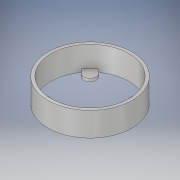
# Autodesk Inventor part: aluminumMount
Saved by Autodesk Inventor 2017 (Build 210142000, 142)
## iProperties
Created: 2016-10-18
Part Number: aluminumMount
Material: Aluminum 6061-AHC
Document SubType Name: Modeling
Designer: cflannery
Density: 2.7 g/cm^3
Appearance: Aluminum - Dark
Author: cflannery
Autodesk Inventor part; units mm, degrees
ref_plane "YZ Plane" through (0, 0, 0) normal (1, 0, 0) x (0, 1, 0)
ref_plane "XZ Plane" through (0, 0, 0) normal (0, 1, 0) x (-1, 0, 0)
ref_plane "XY Plane" through (0, 0, 0) normal (0, 0, 1) x (1, 0, 0)
sketch "Sketch1" plane through (0, 0, 0) normal (0, 1, 0) x (-1, 0, 0)
  circle A0 centre (0, 0) radius 82.55
  circle A1 centre (0, 0) radius 88.9
  dimension "d0" = 165.1
  dimension "d1" = 177.8
  constraints: 2 centre point, 2 coincident
  measures "d0" diameter of A0
  measures "d1" diameter of A1
extrude "Extrusion1" add sketch "Sketch1" along normal blind 50.8
sketch "Sketch2" plane through (0, 0, 0) normal (0, -1, 0) x (1, 0, 0)
  arc A0 (40.4112, 58.3717) -> (58.3717, 40.4112) centre (49.3914, 49.3914) ccw
  arc A1 (58.3717, -40.4112) -> (40.4112, -58.3717) centre (49.3914, -49.3914) ccw
  arc A2 (-40.4112, -58.3717) -> (-58.3717, -40.4112) centre (-49.3914, -49.3914) ccw
  arc A3 (-58.3717, 40.4112) -> (-40.4112, 58.3717) centre (-49.3914, 49.3914) ccw
  circle A4 centre (0, 0) radius 82.55 projected
  line L0 (-40.4112, 58.3717) -> (-48.6965, 66.657)
  line L1 (-58.3717, 40.4112) -> (-66.657, 48.6965)
  line L2 (58.3717, 40.4112) -> (66.657, 48.6965)
  line L3 (40.4112, 58.3717) -> (48.6965, 66.657)
  line L4 (58.3717, -40.4112) -> (66.657, -48.6965)
  line L5 (40.4112, -58.3717) -> (48.6965, -66.657)
  line L6 (-40.4112, -58.3717) -> (-48.6965, -66.657)
  line L7 (-58.3717, -40.4112) -> (-66.657, -48.6965)
  dimension "d4" = 25.4
  constraints: 16 end point, 8 equal length, 8 point on circle, 8 tangent, 4 centre point, 3 equal radius, 2 horizontal alignment, 1 perpendicular, 1 vertical alignment, 13 other
  measures "d4" diameter of A3
extrude "Extrusion2" add sketch "Sketch2" against normal blind 6.35 contours L3 A4 L2 A0 | L0 A3 L1 A4 | A4 L5 A1 L4 | L7 A2 L6 A4
body "Solid1"
